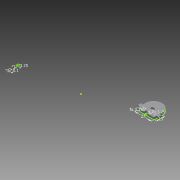
# Autodesk Inventor part: arm-servo
Saved by Autodesk Inventor 2013 (Build 170138000, 138)
## iProperties
Created: 2012-09-08
Part Number: arm-servo
Material: Generic
Document SubType Name: Modeling
Designer: frankenteddy
Density: 1 g/cm^3
Author: frankenteddy
Autodesk Inventor part; units mm, degrees
ref_plane "YZ Plane" through (0, 0, 0) normal (1, 0, 0) x (0, 1, 0)
ref_plane "XZ Plane" through (0, 0, 0) normal (0, 1, 0) x (-1, 0, 0)
ref_plane "XY Plane" through (0, 0, 0) normal (0, 0, 1) x (1, 0, 0)
sketch "Block1" plane through (0, 0, 0) normal (0, 0, 1) x (1, 0, 0)
  circle A0 centre (74.029, 24.2723) radius 1
  line L0 (49.279, 30.4723) -> (71.779, 30.4723)
  line L1 (71.779, 30.4723) -> (71.779, 18.0723)
  line L2 (71.779, 18.0723) -> (49.279, 18.0723)
  line L3 (49.279, 18.0723) -> (49.279, 30.4723)
  line L4 (49.279, 30.4723) -> (44.779, 30.4723)
  line L5 (44.779, 30.4723) -> (44.779, 18.0723)
  line L6 (44.779, 18.0723) -> (49.279, 18.0723)
  line L7 (49.279, 18.0723) -> (49.279, 30.4723)
  line L8 (71.779, 30.4723) -> (76.279, 30.4723)
  line L9 (76.279, 30.4723) -> (76.279, 18.0723)
  line L10 (76.279, 18.0723) -> (71.779, 18.0723)
  line L11 (71.779, 18.0723) -> (71.779, 30.4723)
  line L12 (44.779, 24.2723) -> (76.279, 24.2723) construction
  line L13 (47.029, 30.4723) -> (47.029, 18.0723) construction
  circle A1 centre (47.029, 24.2723) radius 1
  line L14 (74.029, 30.4723) -> (74.029, 18.0723) construction
  point P0 (60.979, 24.0984)
  dimension "d7" = 22.5
  dimension "d8" = 12.4
  dimension "d9" = 4.5
  dimension "d10" = 4.5
  dimension "d11" = 2
  dimension "d12" = 2
  measures "d7" distance of L1.end L2.end
  measures "d8" distance of L0.end L1.end
  measures "d9" distance of L6.end L5.end
  measures "d10" distance of L9.end L10.end
  measures "d11" diameter of A0
  measures "d12" diameter of A1
sketch "Sketch1" plane through (0, 0, 0) normal (0, 0, 1) x (1, 0, 0)
  line L0 (-92.7646, -8.503) -> (-89.7646, -8.503)
  line L1 (-89.7646, -8.503) -> (-89.7646, -11.753)
  line L2 (-89.7646, -11.753) -> (-92.7646, -11.753)
  line L3 (-92.7646, -11.753) -> (-92.7646, -8.503)
  line L4 (-92.7646, -21.6527) -> (-89.7646, -21.6527)
  line L5 (-89.7646, -21.6527) -> (-89.7646, -21.7527)
  line L6 (-89.7646, -21.7527) -> (-92.7646, -21.7527)
  line L7 (-92.7646, -21.7527) -> (-92.7646, -21.6527)
  line L8 (67.7668, 36.0225) -> (94.7668, 36.0225)
  line L9 (94.7668, 36.0225) -> (94.7668, 23.0225)
  line L10 (94.7668, 23.0225) -> (67.7668, 23.0225)
  line L11 (67.7668, 23.0225) -> (67.7668, 36.0225)
  line L12 (67.7668, 29.5225) -> (94.7668, 29.5225) construction
  line L13 (64.5168, 32.0225) -> (67.7668, 32.0225)
  line L14 (67.7668, 32.0225) -> (67.7668, 27.0225)
  line L15 (67.7668, 27.0225) -> (64.5168, 27.0225)
  line L16 (64.5168, 27.0225) -> (64.5168, 32.0225)
  line L17 (64.5168, 29.5225) -> (67.7668, 29.5225) construction
  line L18 (81.2668, 36.0225) -> (81.2668, 23.0225) construction
  line L19 (78.7668, 36.0225) -> (83.7668, 36.0225)
  line L20 (83.7668, 36.0225) -> (83.7668, 32.7725)
  line L21 (83.7668, 32.7725) -> (78.7668, 32.7725)
  line L22 (78.7668, 32.7725) -> (78.7668, 36.0225)
  line L23 (81.2668, 36.0225) -> (81.2668, 32.7725) construction
  line L24 (98.0168, 32.0225) -> (94.7668, 32.0225)
  line L25 (94.7668, 32.0225) -> (94.7668, 27.0225)
  line L26 (94.7668, 27.0225) -> (98.0168, 27.0225)
  line L27 (98.0168, 27.0225) -> (98.0168, 32.0225)
  line L28 (98.0168, 29.5225) -> (94.7668, 29.5225) construction
  line L29 (78.7668, 23.0225) -> (83.7668, 23.0225)
  line L30 (83.7668, 23.0225) -> (83.7668, 26.2725)
  line L31 (83.7668, 26.2725) -> (78.7668, 26.2725)
  line L32 (78.7668, 26.2725) -> (78.7668, 23.0225)
  line L33 (81.2668, 23.0225) -> (81.2668, 26.2725) construction
  arc A0 (94.7668, 36.0225) -> (67.7668, 36.0225) centre (81.2668, 36.0225) ccw
  point P0 (0, 0)
  dimension "d0" = 3
  dimension "mat" = 3.25
  dimension "d2" = 3
  dimension "d3" = 0.1
  dimension "d58" = 27
  dimension "d59" = 13
  dimension "d60" = 3.25
  dimension "d61" = 5
  dimension "d68" = 5
  dimension "d69" = 3.25
  constraints: 68 end point, 14 symmetric about line, 10 parallel, 8 midpoint, 5 horizontal, 5 perpendicular, 4 collinear, 2 point on circle, 2 tangent, 1 centre point
  measures "d0" distance of L1.end L3.start
  measures "mat" distance of L1.start L1.end
  measures "d2" distance of L5.end L7.start
  measures "d3" distance of L5.start L5.end
  measures "d58" distance of L9.end L10.end
  measures "d59" distance of L8.end L9.end
  measures "d60" distance of L14.end L15.end
  measures "d61" distance of L13.end L14.end
  measures "d68" distance of L20.end L21.end
  measures "d69" distance of L19.end L20.end
extrude "Extrusion5" add sketch "Sketch1" along normal blind 3.25 contours L8 L22 L21 L20 L9 L10 L30 L31 L32 L11 | L8 L20 L21 L22 | L11 L15 L16 L13 | L32 L31 L30 L10
extrude "Extrusion7" cut sketch "Sketch1" along normal blind 3.25 contours L8 L20 L21 L22
extrude "Extrusion8" cut sketch "Sketch1" along normal blind 3.25 contours L32 L31 L30 L10
extrude "Extrusion9" add sketch "Sketch1" along normal blind 3.25 contours L24 L27 L26 L9
extrude "Extrusion10" add sketch "Sketch1" along normal blind 3.25 contours A0 L8
equation "\"d60\" = mat"
equation "\"d69\" = mat"
equation "\"d62\" = mat"
equation "\"d70\" = mat"
equation "\"d72\" = mat"
equation "\"d74\" = mat"
equation "\"d76\" = mat"
body "Solid4"
